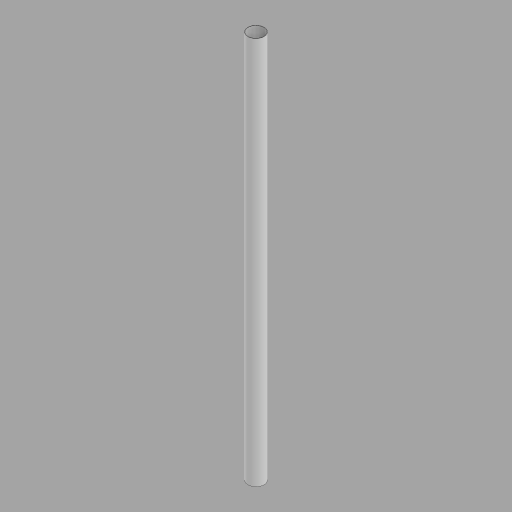
# Autodesk Inventor part: tube
Saved by Autodesk Inventor 2024 (Build 280153020, 153B)
## iProperties
Created: 2023-10-26
Part Number: tube
Material: Generic
Document SubType Name: Modeling
Designer: schanen
Density: 1 g/cm^3
Appearance: Default
Mass: 4.96566 g
Surface Area: 397.659 cm^2
Volume: 4.96566 cm^3
tube_od: 12.700 mm
tube_wall: 0.254 mm
Author: schanen
Autodesk Inventor part; units mm, degrees
ref_plane "XZ Plane" through (0, 0, 0) normal (0, 1, 0) x (-1, 0, 0)
ref_plane "XY Plane" through (0, 0, 0) normal (0, 0, 1) x (1, 0, 0)
sketch "Sketch1" plane through (0, 0, 0) normal (0, 1, 0) x (-1, 0, 0)
  circle A0 centre (0, 0) radius 6.35
  circle A1 centre (0, 0) radius 6.096
  dimension "tube_od" = 12.7
  dimension "tube_wall" = 0.254
  constraints: 2 centre point, 2 coincident
  measures "tube_od" diameter of A0
  measures "tube_wall" radial gap between concentric circles of A0 A1
extrude "Extrusion1" add sketch "Sketch1" along normal blind 300
ref_plane "Work Plane1" through (6, 0, 0) normal (1, 0, 0) x (0, 1, 0)
sketch "Sketch2" plane through (6, 0, 0) normal (1, 0, 0) x (0, 1, 0)
  line L0 (0, -6.35) -> (0, 6.35) projected
  line L1 (300, -6.35) -> (300, 6.35) projected
  point P0 (0, 0)
  point P1 (150, 0)
  point P2 (0, 0)
  dimension "d5" = 300
  dimension "d6" = 150
  constraints: 1 horizontal alignment, 1 midpoint
  measures "d5" distance between parallel lines of L0 L1
  measures "d6" distance of point (0, 0) point (150, 0)
hole "Hole1" [suppressed]
pattern_linear "Rectangular Pattern1" [suppressed]
equation "\"d6\" = 0.5 * d5"
body "Solid1"
